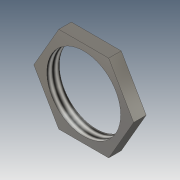
# Autodesk Inventor part: Porca da Chave Seletora
Saved by Autodesk Inventor 2016 (Build 200138000, 138)
## iProperties
Created: 2018-12-09
Part Number: Porca da Chave Seletora
Material: Generic
Document SubType Name: Modeling
Designer: Pedro Mendonça
Density: 1 g/cm^3
Appearance: Steel - Polished
Author: Pedro Mendonça
Autodesk Inventor part; units mm, degrees
ref_plane "YZ Plane" through (0, 0, 0) normal (1, 0, 0) x (0, 1, 0)
ref_plane "XZ Plane" through (0, 0, 0) normal (0, 1, 0) x (-1, 0, 0)
ref_plane "XY Plane" through (0, 0, 0) normal (0, 0, 1) x (1, 0, 0)
sketch "Sketch1" plane through (0, 0, 0) normal (1, 0, 0) x (0, 1, 0)
  line L0 (7.9674, 0) -> (3.9837, -6.9)
  line L1 (3.9837, -6.9) -> (-3.9837, -6.9)
  line L2 (-3.9837, -6.9) -> (-7.9674, 0)
  line L3 (-7.9674, 0) -> (-3.9837, 6.9)
  line L4 (-3.9837, 6.9) -> (3.9837, 6.9)
  line L5 (3.9837, 6.9) -> (7.9674, 0)
  circle A0 centre (0, 0) radius 5.9
  dimension "d0" = 13.8
  dimension "d1" = 11.8
  constraints: 12 end point, 2 coincident, 1 centre point, 13 other
  measures "d0" distance between parallel lines of L1 L4
  measures "d1" diameter of A0
extrude "Extrusion1" add sketch "Sketch1" along normal mid plane 2
thread "Thread1" size "M12x1" class "6H" standard "ANSI Metric M Profile" full length
body "Solid1"
